Autodesk Fusion 360 part; units mm, degrees
(part 2 of 2)
sketch "Sketch2" plane through (0, 0, 0) normal (0, -1, 0) x (1, 0, 0)
  line L0 (6, -13.1754) -> (3.25, -11.5877)
  line L1 (3.25, -11.5877) -> (3.25, -8.4123)
  line L2 (3.25, -8.4123) -> (6, -6.8246)
  line L3 (6, -6.8246) -> (8.75, -8.4123)
  line L4 (8.75, -8.4123) -> (8.75, -11.5877)
  line L5 (8.75, -11.5877) -> (6, -13.1754)
  line L6 (165.75, -33.5877) -> (163, -35.1754)
  line L7 (163, -35.1754) -> (160.25, -33.5877)
  line L8 (160.25, -33.5877) -> (160.25, -30.4123)
  line L9 (160.25, -30.4123) -> (163, -28.8246)
  line L10 (163, -28.8246) -> (165.75, -30.4123)
  line L11 (165.75, -30.4123) -> (165.75, -33.5877)
  line L12 (37, -243.1754) -> (34.25, -241.5877)
  line L13 (34.25, -241.5877) -> (34.25, -238.4123)
  line L14 (34.25, -238.4123) -> (37, -236.8246)
  line L15 (37, -236.8246) -> (39.75, -238.4123)
  line L16 (39.75, -238.4123) -> (39.75, -241.5877)
  line L17 (39.75, -241.5877) -> (37, -243.1754)
  line L18 (191.25, -219.5877) -> (191.25, -216.4123)
  line L19 (191.25, -216.4123) -> (194, -214.8246)
  line L20 (194, -214.8246) -> (196.75, -216.4123)
  line L21 (196.75, -216.4123) -> (196.75, -219.5877)
  line L22 (196.75, -219.5877) -> (194, -221.1754)
  line L23 (194, -221.1754) -> (191.25, -219.5877)
  line L24 (163, -214.8246) -> (165.75, -216.4123)
  line L25 (165.75, -216.4123) -> (165.75, -219.5877)
  line L26 (165.75, -219.5877) -> (163, -221.1754)
  line L27 (163, -221.1754) -> (160.25, -219.5877)
  line L28 (160.25, -219.5877) -> (160.25, -216.4123)
  line L29 (160.25, -216.4123) -> (163, -214.8246)
  line L30 (39.75, -219.5877) -> (37, -221.1754)
  line L31 (37, -221.1754) -> (34.25, -219.5877)
  line L32 (34.25, -219.5877) -> (34.25, -216.4123)
  line L33 (34.25, -216.4123) -> (37, -214.8246)
  line L34 (37, -214.8246) -> (39.75, -216.4123)
  line L35 (39.75, -216.4123) -> (39.75, -219.5877)
  line L36 (194, -6.8246) -> (196.75, -8.4123)
  line L37 (196.75, -8.4123) -> (196.75, -11.5877)
  line L38 (196.75, -11.5877) -> (194, -13.1754)
  line L39 (194, -13.1754) -> (191.25, -11.5877)
  line L40 (191.25, -11.5877) -> (191.25, -8.4123)
  line L41 (191.25, -8.4123) -> (194, -6.8246)
  line L42 (37, -13.1754) -> (34.25, -11.5877)
  line L43 (34.25, -11.5877) -> (34.25, -8.4123)
  line L44 (34.25, -8.4123) -> (37, -6.8246)
  line L45 (37, -6.8246) -> (39.75, -8.4123)
  line L46 (39.75, -8.4123) -> (39.75, -11.5877)
  line L47 (39.75, -11.5877) -> (37, -13.1754)
  line L48 (3.25, -30.4123) -> (6, -28.8246)
  line L49 (6, -28.8246) -> (8.75, -30.4123)
  line L50 (8.75, -30.4123) -> (8.75, -33.5877)
  line L51 (8.75, -33.5877) -> (6, -35.1754)
  line L52 (6, -35.1754) -> (3.25, -33.5877)
  line L53 (3.25, -33.5877) -> (3.25, -30.4123)
  line L54 (191.25, -30.4123) -> (194, -28.8246)
  line L55 (194, -28.8246) -> (196.75, -30.4123)
  line L56 (196.75, -30.4123) -> (196.75, -33.5877)
  line L57 (196.75, -33.5877) -> (194, -35.1754)
  line L58 (194, -35.1754) -> (191.25, -33.5877)
  line L59 (191.25, -33.5877) -> (191.25, -30.4123)
  line L60 (3.25, -238.4123) -> (6, -236.8246)
  line L61 (6, -236.8246) -> (8.75, -238.4123)
  line L62 (8.75, -238.4123) -> (8.75, -241.5877)
  line L63 (8.75, -241.5877) -> (6, -243.1754)
  line L64 (6, -243.1754) -> (3.25, -241.5877)
  line L65 (3.25, -241.5877) -> (3.25, -238.4123)
  line L66 (194, -243.1754) -> (191.25, -241.5877)
  line L67 (191.25, -241.5877) -> (191.25, -238.4123)
  line L68 (191.25, -238.4123) -> (194, -236.8246)
  line L69 (194, -236.8246) -> (196.75, -238.4123)
  line L70 (196.75, -238.4123) -> (196.75, -241.5877)
  line L71 (196.75, -241.5877) -> (194, -243.1754)
  line L72 (165.75, -238.4123) -> (165.75, -241.5877)
  line L73 (165.75, -241.5877) -> (163, -243.1754)
  line L74 (163, -243.1754) -> (160.25, -241.5877)
  line L75 (160.25, -241.5877) -> (160.25, -238.4123)
  line L76 (160.25, -238.4123) -> (163, -236.8246)
  line L77 (163, -236.8246) -> (165.75, -238.4123)
  line L78 (8.75, -219.5877) -> (6, -221.1754)
  line L79 (6, -221.1754) -> (3.25, -219.5877)
  line L80 (3.25, -219.5877) -> (3.25, -216.4123)
  line L81 (3.25, -216.4123) -> (6, -214.8246)
  line L82 (6, -214.8246) -> (8.75, -216.4123)
  line L83 (8.75, -216.4123) -> (8.75, -219.5877)
  line L84 (160.25, -11.5877) -> (160.25, -8.4123)
  line L85 (160.25, -8.4123) -> (163, -6.8246)
  line L86 (163, -6.8246) -> (165.75, -8.4123)
  line L87 (165.75, -8.4123) -> (165.75, -11.5877)
  line L88 (165.75, -11.5877) -> (163, -13.1754)
  line L89 (163, -13.1754) -> (160.25, -11.5877)
  line L90 (39.75, -30.4123) -> (39.75, -33.5877)
  line L91 (39.75, -33.5877) -> (37, -35.1754)
  line L92 (37, -35.1754) -> (34.25, -33.5877)
  line L93 (34.25, -33.5877) -> (34.25, -30.4123)
  line L94 (34.25, -30.4123) -> (37, -28.8246)
  line L95 (37, -28.8246) -> (39.75, -30.4123)
  line L96 (0, 0) -> (0, -250)
  line L97 (0, -250) -> (200, -250)
  line L98 (200, -250) -> (200, 0)
  line L99 (200, 0) -> (0, 0)
  circle A0 centre (160, -60) radius 2
  circle A1 centre (116, -60) radius 2
  circle A2 centre (160, -100) radius 2
  circle A3 centre (116, -100) radius 2
  circle A4 centre (50, -15) radius 2
  circle A5 centre (88, -15) radius 2
  circle A6 centre (87.486, -53) radius 2
  circle A7 centre (49.486, -52.9965) radius 2
  circle A8 centre (50, -67.9965) radius 2
  circle A9 centre (88, -68) radius 2
  circle A10 centre (88, -106) radius 2
  circle A11 centre (50, -105.9965) radius 2
  circle A12 centre (150, -215) radius 2
  circle A13 centre (100, -215) radius 2
  circle A14 centre (150, -157) radius 2
  circle A15 centre (100, -157) radius 2
  line L100 (118.75, -61.5877) -> (118.75, -58.4123)
  line L101 (118.75, -58.4123) -> (116, -56.8246)
  line L102 (116, -56.8246) -> (113.25, -58.4123)
  line L103 (113.25, -58.4123) -> (113.25, -61.5877)
  line L104 (113.25, -61.5877) -> (116, -63.1754)
  line L105 (116, -63.1754) -> (118.75, -61.5877)
  line L106 (162.75, -61.5877) -> (162.75, -58.4123)
  line L107 (162.75, -58.4123) -> (160, -56.8246)
  line L108 (160, -56.8246) -> (157.25, -58.4123)
  line L109 (157.25, -58.4123) -> (157.25, -61.5877)
  line L110 (157.25, -61.5877) -> (160, -63.1754)
  line L111 (160, -63.1754) -> (162.75, -61.5877)
  line L112 (118.75, -101.5877) -> (118.75, -98.4123)
  line L113 (118.75, -98.4123) -> (116, -96.8246)
  line L114 (116, -96.8246) -> (113.25, -98.4123)
  line L115 (113.25, -98.4123) -> (113.25, -101.5877)
  line L116 (113.25, -101.5877) -> (116, -103.1754)
  line L117 (116, -103.1754) -> (118.75, -101.5877)
  line L118 (160, -103.1754) -> (162.75, -101.5877)
  line L119 (162.75, -101.5877) -> (162.75, -98.4123)
  line L120 (162.75, -98.4123) -> (160, -96.8246)
  line L121 (160, -96.8246) -> (157.25, -98.4123)
  line L122 (157.25, -98.4123) -> (157.25, -101.5877)
  line L123 (157.25, -101.5877) -> (160, -103.1754)
  point P0 (116, -60)
  point P1 (160, -60)
  point P2 (116, -100)
  point P3 (160, -100)
  dimension "d25" = 4
  dimension "d26" = 60
  dimension "d27" = 4
  dimension "d28" = 60
  dimension "d29" = 44
  dimension "d30" = 40
  dimension "d31" = 4
  dimension "d32" = 4
  dimension "d33" = 40
  dimension "d34" = 40
  dimension "d35" = 44
  dimension "d36" = 40
  dimension "d37" = 4
  dimension "d38" = 4
  dimension "d39" = 15
  dimension "d40" = 15
  dimension "d41" = 50
  dimension "d42" = 38
  dimension "d43" = 4
  dimension "d44" = 4
  dimension "d45" = 38
  dimension "d46" = 38
  dimension "d47" = 38
  dimension "d48" = 4
  dimension "d49" = 4
  dimension "d50" = 4
  dimension "d51" = 4
  dimension "d52" = 38
  dimension "d53" = 38
  dimension "d54" = 50
  dimension "d55" = 50
  dimension "d56" = 38
  dimension "d57" = 38
  dimension "d58" = 15
  dimension "d60" = 15
  dimension "d61" = 4
  dimension "d62" = 4
  dimension "d63" = 4
  dimension "d64" = 4
  dimension "d65" = 50
  dimension "d66" = 50
  dimension "d67" = 58
  dimension "d68" = 58
  dimension "d69" = 50
  dimension "d70" = 50
  dimension "d71" = 35
  dimension "d74" = 2.75
  dimension "d75" = 2.75
  dimension "d76" = 2.75
  dimension "d77" = 2.75
  constraint coincident P0 A1.centre
  constraint coincident P1 A0.centre
  constraint coincident P2 A3.centre
  constraint coincident P3 A2.centre
  constraint parallel L98 L106
  constraint parallel L98 L119
  constraint parallel L100 L109
  constraint parallel L112 L122
  measures "d25" diameter of A0
  measures "d26" distance of L99 P1
  measures "d27" diameter of A1
  measures "d28" distance of L99 P0
  measures "d29" distance of P1 P0
  measures "d30" distance of L98 P1
  measures "d31" diameter of A2
  measures "d32" diameter of A3
  measures "d33" vertical distance of P1 P3
  measures "d34" vertical distance of P0 P2
  measures "d35" distance of P3 P2
  measures "d36" distance of L98 P3
  measures "d37" diameter of A4
  measures "d38" diameter of A5
  measures "d39" distance of L99 A5.centre
  measures "d40" distance of L99 A4.centre
  measures "d41" distance of L96 A4.centre
  measures "d42" distance of A4.centre A5.centre
  measures "d43" diameter of A6
  measures "d44" diameter of A7
  measures "d45" vertical distance of A5.centre A6.centre
  measures "d46" horizontal distance of A6.centre A7.centre
  measures "d47" distance of A4.centre A7.centre
  measures "d48" diameter of A8
  measures "d49" diameter of A9
  measures "d50" diameter of A10
  measures "d51" diameter of A11
  measures "d52" horizontal distance of A8.centre A9.centre
  measures "d53" horizontal distance of A10.centre A11.centre
  measures "d54" distance of L96 A8.centre
  measures "d55" distance of L96 A11.centre
  measures "d56" distance of A8.centre A11.centre
  measures "d57" distance of A9.centre A10.centre
  measures "d58" vertical distance of A7.centre A8.centre
  measures "d60" vertical distance of A6.centre A9.centre
  measures "d61" diameter of A12
  measures "d62" diameter of A13
  measures "d63" diameter of A14
  measures "d64" diameter of A15
  measures "d65" horizontal distance of A12.centre A13.centre
  measures "d66" distance of A14.centre A15.centre
  measures "d67" vertical distance of A12.centre A14.centre
  measures "d68" vertical distance of A13.centre A15.centre
  measures "d69" distance of L98 A12.centre
  measures "d70" distance of L98 A14.centre
  measures "d71" distance of L97 A12.centre
  measures "d74" distance of P0 L105
  measures "d75" distance of P1 L111
  measures "d76" distance of P2 L117
  measures "d77" distance of P3 L123
extrude "Extrude3" cut sketch "Sketch2" against normal blind 40 contours A0 | A1 | A2 | A3 | A4 | A5 | A6 | A7 | A8 | A9 | A10 | A11 | A12 | A13 | A14 | A15
extrude "Extrude4" cut sketch "Sketch2" along normal blind 2.4 from surface at -5 contours L100 L101 L102 L103 L104 L105 | L106 L107 L108 L109 L110 L111 | L112 L113 L114 L115 L116 L117 | L118 L119 L120 L121 L122 L123

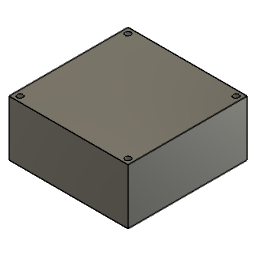
design "Pont en H"
Autodesk Fusion 360 part; units mm, degrees
sketch "Sketch1" plane through (0, 0, 0) normal (0, 1, 0) x (1, 0, 0)
  line L0 (-20, 20) -> (23, 20)
  line L1 (23, 20) -> (23, -23)
  line L2 (23, -23) -> (-20, -23)
  line L3 (-20, -23) -> (-20, 20)
  dimension "d1" = 43
  dimension "d2" = 43
  constraint horizontal L0
  constraint vertical L1
  constraint horizontal L2
  constraint vertical L3
  measures "d1" distance of L0.start L0.end
  measures "d2" distance of L0.start L2.end
extrude "Extrude1" add sketch "Sketch1" along normal blind 20
sketch "Sketch3" plane through (0, 20, 0) normal (0, 1, 0) x (-1, 0, 0)
  line L0 (20, 23) -> (-23, 23)
  line L1 (-23, 23) -> (-23, -20)
  line L2 (-23, -20) -> (20, -20)
  line L3 (20, -20) -> (20, 23)
  circle A0 centre (18, -18) radius 1
  line L4 (-1.5, -20) -> (-1.5, 23)
  circle A1 centre (-21, -18) radius 1
  line L5 (20, 1.5) -> (-23, 1.5)
  circle A2 centre (18, 21) radius 1
  circle A3 centre (-21, 21) radius 1
  dimension "d5" = 2
  dimension "d6" = 2
  dimension "d7" = 2
  constraint midpoint L2 L4.start
  constraint midpoint L0 L4.end
  constraint symmetric A0 L4 A1
  constraint midpoint L3 L5.start
  constraint midpoint L1 L5.end
  constraint symmetric A0 L5 A2
  constraint symmetric A1 L5 A3
  measures "d5" diameter of A0
  measures "d6" distance of L2 A0.centre
  measures "d7" distance of L3 A0.centre
extrude "Extrude2" cut sketch "Sketch3" against normal blind 30 contours A0 | A1 | A2 | A3

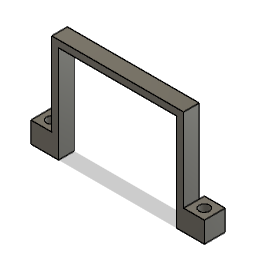
design "fixation batterie"
Autodesk Fusion 360 part; units mm, degrees
sketch "Sketch1" plane through (0, 0, 0) normal (0, 0, 1) x (1, 0, 0)
  line L0 (0, 0) -> (6, 0)
  line L1 (6, 0) -> (6, 6)
  line L2 (6, 6) -> (0, 6)
  line L3 (0, 6) -> (0, 0)
  line L4 (6, 0) -> (8, 0)
  line L5 (8, 0) -> (8, 30)
  line L6 (8, 30) -> (6, 30)
  line L7 (6, 30) -> (6, 0)
  line L8 (6, 30) -> (25, 30)
  line L9 (25, 30) -> (25, 28)
  line L10 (25, 28) -> (6, 28)
  line L11 (6, 28) -> (6, 30)
  line L12 (50, 6) -> (50, 0)
  line L13 (44, 6) -> (50, 6)
  line L14 (44, 0) -> (42, 0)
  line L15 (50, 0) -> (44, 0)
  line L16 (44, 30) -> (25, 30)
  line L17 (42, 0) -> (42, 30)
  line L18 (44, 0) -> (44, 6)
  line L19 (44, 30) -> (44, 0)
  line L20 (25, 28) -> (44, 28)
  line L21 (44, 28) -> (44, 30)
  line L22 (42, 30) -> (44, 30)
  point P0 (50, 0)
  dimension "d1" = 6
  dimension "d2" = 6
  dimension "d3" = 2
  dimension "d4" = 30
  dimension "d5" = 19
  dimension "d6" = 2
  constraint horizontal L0
  constraint vertical L1
  constraint horizontal L2
  constraint vertical L3
  constraint coincident L0.start L3.end
  constraint horizontal L4
  constraint vertical L5
  constraint horizontal L6
  constraint vertical L7
  constraint horizontal L8
  constraint vertical L9
  constraint horizontal L10
  constraint vertical L11
  constraint symmetric L0.start L9 L12.end
  constraint symmetric L0.start L9 P0
  constraint symmetric L0.end L9 L14.start
  constraint symmetric L1.end L9 L13.start
  constraint symmetric L2.end L9 L12.start
  constraint symmetric L4.end L9 L14.end
  constraint symmetric L5.end L9 L17.end
  constraint symmetric L6.end L9 L16.start
  constraint symmetric L8.end L9 L16.end
  constraint symmetric L10.start L9 L20.start
  constraint symmetric L10.end L9 L20.end
  measures "d1" distance of L0.start L0.end
  measures "d2" distance of L0.start L2.end
  measures "d3" distance of L0.end L4.end
  measures "d4" distance of L0.end L6.end
  measures "d5" distance of L6.end L8.end
  measures "d6" distance of L6.end L10.end
extrude "Extrude1" add sketch "Sketch1" along normal blind 3 and the other way blind 3 contours L0 L1 L2 L3 L7 | L12 L13 L15 L18 L19 makes body 1 at (0, 2, 1) makes body 2 at (46, 2, 3)
extrude "Extrude2" add sketch "Sketch1" along normal blind 1.5 and the other way blind 1.5 contours L1 L4 L5 L7 L10 | L5 L6 L7 L8 L10 L11 | L5 L8 L9 L10 | L9 L16 L17 L20 | L14 L17 L18 L19 L20 | L16 L17 L19 L20 L21 L22 bodies 1 2
sketch "Sketch2" plane through (0, 6, 0) normal (0, 1, 0) x (-1, 0, 0)
  line L0 (0, -3) -> (0, 3)
  line L1 (0, 3) -> (-6, 3)
  line L2 (-6, 3) -> (-6, 1.5)
  line L3 (-6, 1.5) -> (-6, -1.5)
  line L4 (-6, -1.5) -> (-6, -3)
  line L5 (-6, -3) -> (0, -3)
  circle A0 centre (-3, 0) radius 1.5
  circle A1 centre (-47, 0) radius 1.5
  line L6 (-50, -3) -> (-50, 3)
  line L7 (-44, -3) -> (-50, -3)
  dimension "d15" = 3
  dimension "d16" = 3
  dimension "d17" = 3
  dimension "d18" = 3
  dimension "d19" = 3
  dimension "d20" = 3
  measures "d15" diameter of A1
  measures "d16" diameter of A0
  measures "d17" distance of L5 A0.centre
  measures "d18" distance of L0 A0.centre
  measures "d19" distance of A1.centre L6
  measures "d20" distance of A1.centre L7
extrude "Extrude3" cut sketch "Sketch2" against normal blind 18 contours A0 | A1 bodies 1
extrude "Extrude4" add 1 faces at (7.3333, 11.3333, 1.5) along direction (0, 0, 1) blind 1.5 on bodies 1 bodies 1

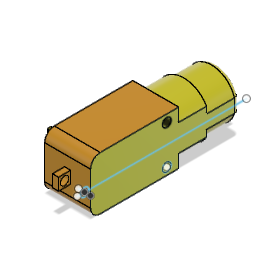
design "moto reducteur"
Autodesk Fusion 360 part; units mm, degrees
sketch "Sketch1" plane through (0, 0, 0) normal (0, 0, 1) x (1, 0, 0)
  line L0 (0, 0) -> (19, 0)
  line L1 (19, 0) -> (19, 22)
  line L2 (19, 22) -> (0, 22)
  line L3 (0, 22) -> (0, 0)
  line L4 (0, 22) -> (19, 0)
  line L5 (19, 22) -> (0, 0)
  arc A0 (0, 5.4547) -> (19, 5.4547) centre (9.5, 11) ccw
  arc A1 (19, 16.5453) -> (0, 16.5453) centre (9.5, 11) ccw
  dimension "d1" = 19
  dimension "d2" = 22
  constraint horizontal L0
  constraint vertical L1
  constraint horizontal L2
  constraint vertical L3
  constraint coincident L0.start L3.end
  constraint midpoint L4 A0.centre
  constraint tangent L2 A0
  constraint coincident L3 A1.end
  constraint coincident L3 A0.start
  constraint coincident L1 A0.end
  constraint coincident L1 A1.start
  constraint concentric A0 A1
  measures "d1" distance of L0.start L0.end
  measures "d2" distance of L0.start L2.end
extrude "Extrude1" add sketch "Sketch1" along normal blind 36.5
extrude "Extrude2" add sketch "Sketch1" against normal blind 11.5 contours L4 L5 A0 | L3 L4 L5 A0 A1 | L1 L4 L5 A0 A1 | L4 L5 A1
sketch "Sketch2" plane through (0, 0, -11.5) normal (0, 0, -1) x (-1, 0, 0)
  arc A0 (0, 16.5453) -> (-19, 16.5453) centre (-9.5, 11) ccw
  line L0 (-19, 16.5453) -> (-19, 5.4547)
  arc A1 (-19, 5.4547) -> (0, 5.4547) centre (-9.5, 11) ccw
  line L1 (0, 5.4547) -> (0, 16.5453)
  arc A2 (-19, 8.2143) -> (0, 8.2143) centre (-9.5, 11) ccw
  arc A3 (0, 13.7857) -> (-19, 13.7857) centre (-9.5, 11) ccw
  line L2 (-19, 13.7857) -> (-19, 8.2143)
  line L3 (0, 13.7857) -> (0, 8.2143)
  dimension "d7" = 19.8
  constraint concentric A0 A2
  constraint coincident L0 A3.end
  constraint coincident L0 A2.start
  constraint coincident L1 A2.end
  constraint coincident L1 A3.start
  constraint concentric A2 A3
  measures "d7" diameter of A2
extrude "Extrude3" add sketch "Sketch2" along normal blind 13.5 contours L0 L1 A2 A3 L2 L3
sketch "Sketch3" plane through (0, 0, 0) normal (-1, 0, 0) x (0, 0, 1)
  line L0 (0, 22) -> (0, 16.5453)
  line L1 (0, 16.5453) -> (-11.5, 16.5453)
  line L2 (-11.5, 16.5453) -> (-11.5, 13.7857)
  line L3 (-11.5, 13.7857) -> (-25, 13.7857)
  line L4 (-25, 13.7857) -> (-25, 8.2143)
  line L5 (-25, 8.2143) -> (-11.5, 8.2143)
  line L6 (-11.5, 8.2143) -> (-11.5, 5.4547)
  line L7 (-11.5, 5.4547) -> (0, 5.4547)
  line L8 (0, 5.4547) -> (0, 0)
  line L9 (0, 0) -> (36.5, 0)
  line L10 (36.5, 0) -> (36.5, 22)
  line L11 (36.5, 22) -> (0, 22)
  line L12 (36.5, 0) -> (14.5, 0)
  line L13 (14.5, 0) -> (14.5, 22)
  line L14 (14.5, 22) -> (36.5, 22)
  line L15 (36.5, 22) -> (36.5, 0)
  line L16 (14.5, 22) -> (36.5, 0)
  line L17 (36.5, 22) -> (14.5, 0)
  line L18 (24.625, 8.6581) -> (24.625, 13.3419)
  line L19 (26.375, 13.3419) -> (26.375, 8.6581)
  line L20 (26.375, 8.6581) -> (24.625, 13.3419) construction
  line L21 (24.625, 8.6581) -> (26.375, 13.3419) construction
  arc A0 (24.625, 8.6581) -> (26.375, 8.6581) centre (25.5, 11) ccw
  arc A1 (26.375, 13.3419) -> (24.625, 13.3419) centre (25.5, 11) ccw
  circle A2 centre (25.5, 11) radius 2.75
  circle A3 centre (25.5, 11) radius 3
  point P0 (25.5, 11)
  dimension "d10" = 22
  dimension "d11" = 22
  dimension "d12" = 5
  dimension "d13" = 1.75
  dimension "d39" = 5.5
  dimension "d40" = 6
  constraint horizontal L12
  constraint vertical L13
  constraint horizontal L14
  constraint vertical L15
  constraint coincident L9.end L10.start
  constraint coincident L10.end L11.start
  constraint midpoint L16 P0
  constraint parallel L18 L19
  constraint coincident L20 P0
  constraint coincident L21 P0
  constraint coincident P0 A0.centre
  constraint concentric A0 A1
  constraint concentric A0 A2
  measures "d10" distance of L9.end L12.end
  measures "d11" distance of L9.end L10.end
  measures "d12" diameter of A0
  measures "d13" distance of L18.end L19.start
  measures "d39" diameter of A2
  measures "d40" diameter of A3
sketch "Sketch4" plane through (0, 0, -25) normal (0, 0, -1) x (-1, 0, 0)
  line L0 (-19, 13.7857) -> (-19, 8.2143)
  arc A0 (-19, 8.2143) -> (0, 8.2143) centre (-9.5, 11) ccw
  line L1 (0, 8.2143) -> (0, 13.7857)
  arc A1 (0, 13.7857) -> (-19, 13.7857) centre (-9.5, 11) ccw
  circle A2 centre (-9.5, 11) radius 4.75
  dimension "d14" = 9.5
  constraint concentric A0 A2
  measures "d14" diameter of A2
extrude "Extrude4" add sketch "Sketch4" along normal blind 2.5 contours A2
extrude "Extrude5" add sketch "Sketch3" along normal blind 9 contours L16 L17 L18 L19 A1 | L16 L17 L18 | L16 L17 L19 | L16 L17 L18 L19 A0
sketch "Sketch5" plane through (0, 0, 36.5) normal (0, 0, 1) x (1, 0, 0)
  line L0 (0, 22) -> (0, 0)
  line L1 (0, 0) -> (19, 0)
  line L2 (19, 0) -> (19, 22)
  line L3 (19, 22) -> (0, 22)
  line L4 (0, 22) -> (19, 0)
  line L5 (10.75, 13.5) -> (8.25, 13.5)
  line L6 (8.25, 13.5) -> (8.25, 8.5)
  line L7 (8.25, 8.5) -> (10.75, 8.5)
  line L8 (10.75, 8.5) -> (10.75, 13.5)
  line L9 (10.75, 13.5) -> (8.25, 8.5) construction
  line L10 (8.25, 13.5) -> (10.75, 8.5) construction
  point P0 (9.5, 11)
  dimension "d19" = 2.5
  dimension "d20" = 5
  constraint coincident L0.start L3.end
  constraint coincident L1.end L2.start
  constraint horizontal L5
  constraint perpendicular L5 L6
  constraint parallel L5 L7
  constraint parallel L6 L8
  constraint coincident L9 P0
  constraint coincident L10 P0
  constraint midpoint L4 P0
  measures "d19" distance of L6.end L7.end
  measures "d20" distance of L5.end L6.end
extrude "Extrude6" add sketch "Sketch5" along normal blind 5 contours L4 L5 L6 L8 | L4 L6 L7 L8
sketch "Sketch6" plane through (0, 0, -27.5) normal (0, 0, -1) x (-1, 0, 0)
  circle A0 centre (-9.5, 11) radius 4.75
  circle A1 centre (-9.5, 11) radius 0.9
  dimension "d23" = 1.8
  constraint concentric A0 A1
  measures "d23" diameter of A1
extrude "Extrude7" add sketch "Sketch6" along normal blind 0.1 contours A1
fillet "Fillet1" radius 0.9 1 edges at (10.3391, 10.6745, -27.6)
fillet "Fillet2" radius 2 4 edges at (9.5, 20.9, -25) (9.5, 1.1, -25) (19, 11, -25) (0, 11, -25)
fillet "Fillet3" radius 4 2 edges at (9.5, 22, 36.5) (9.5, 0, 36.5)
sketch "Sketch7" plane through (19, 0, 0) normal (1, 0, 0) x (0, 0, -1)
  arc A0 (-36.5, 4) -> (-32.5, 0) centre (-32.5, 4) ccw
  line L0 (-32.5, 0) -> (0, 0)
  line L1 (0, 0) -> (0, 5.4547)
  line L2 (0, 5.4547) -> (11.5, 5.4547)
  line L3 (11.5, 5.4547) -> (11.5, 8.2143)
  line L4 (11.5, 8.2143) -> (23, 8.2143)
  line L5 (23, 8.2143) -> (23, 13.7857)
  line L6 (23, 13.7857) -> (11.5, 13.7857)
  line L7 (11.5, 13.7857) -> (11.5, 16.5453)
  line L8 (11.5, 16.5453) -> (0, 16.5453)
  line L9 (0, 16.5453) -> (0, 22)
  line L10 (0, 22) -> (-32.5, 22)
  arc A1 (-32.5, 22) -> (-36.5, 18) centre (-32.5, 18) ccw
  line L11 (-36.5, 18) -> (-36.5, 4)
  circle A2 centre (-5, 19) radius 1.75
  line L12 (-42, 11) -> (28, 11)
  circle A3 centre (-5, 3) radius 1.75
  line L13 (-41.5, 13.5) -> (-36.5, 8.4999)
  circle A4 centre (-39, 10.9999) radius 1.75
  dimension "d32" = 3.5
  dimension "d33" = 3
  dimension "d34" = 5
  dimension "d38" = 3.5
  constraint perpendicular L5 L12
  constraint symmetric A2 L12 A3
  constraint coincident L11 L13.end
  constraint midpoint L13 A4.centre
  measures "d32" diameter of A2
  measures "d33" distance of L10 A2.centre
  measures "d34" distance of L9 A2.centre
  measures "d38" diameter of A4
extrude "Extrude8" cut sketch "Sketch7" against normal blind 20 contours L12 L13 A4 | L12 L13 A4 | L12 L13 A4 | L12 L13 A4 | A2 | A3
extrude "Extrude9" cut sketch "Sketch3" against normal blind 18 contours L16 L17 A2 A3 | L16 L17 A2 A3 | L16 L17 A2 A3 | L16 L17 A2 A3
